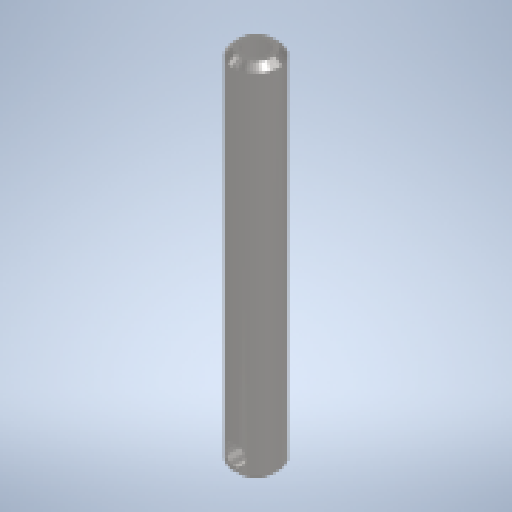
# Autodesk Inventor part: part5
Saved by Autodesk Inventor 2025.2 (Build 292293000, 293)
## iProperties
Created: 2024-12-08
Part Number: part5
Material: Stal nierdzewna
Document SubType Name: Modeling
Designer: Marek
Density: 8 g/cm^3
Appearance: Częściowo polerowany
Author: Marek
Autodesk Inventor part; units mm, degrees
ref_plane "YZ Plane" through (0, 0, 0) normal (1, 0, 0) x (0, 1, 0)
ref_plane "XZ Plane" through (0, 0, 0) normal (0, 1, 0) x (-1, 0, 0)
ref_plane "XY Plane" through (0, 0, 0) normal (0, 0, 1) x (1, 0, 0)
sketch "Szkic1" plane through (0, 0, 0) normal (0, 1, 0) x (-1, 0, 0)
  circle A0 centre (0, 0) radius 5.7
  dimension "d0" = 11.4
  constraints: 1 centre point, 1 coincident
  measures "d0" diameter of A0
extrude "Wyciągnięcie proste1" add sketch "Szkic1" along normal blind 90
sketch "Szkic5" plane through (0, 90, 0) normal (0, 1, 0) x (1, 0, 0)
  point P0 (0, 0)
  point P1 (0, 0)
hole "Otwór2" at (0, 90, 0) direction (0, -1, 0) diameter 6 depth 35 tip angle 120
chamfer "Faza1" distance 1.5 angle 45 2 edges at (5.7, 90, 0) (5.7, 0, 0)
sketch "Szkic6" plane through (0, 0, 0) normal (0, 0, 1) x (1, 0, 0)
  circle A0 centre (0, 5) radius 2.5
  point P0 (0, 0)
  dimension "d20" = 5
  constraints: 1 centre point
  measures "d20" diameter of A0
extrude "Wyciągnięcie proste2" cut sketch "Szkic6" along normal mid plane 30
